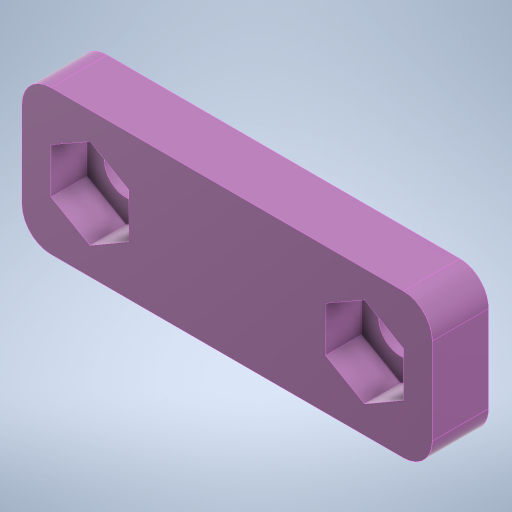
# Autodesk Inventor part: Крепежи динамиков
Saved by Autodesk Inventor 2024 (Build 280153020, 153B)
## iProperties
Created: 2023-06-10
Part Number: Крепежи динамиков
Material: Типовые
Document SubType Name: Modeling
Designer: Admin
Density: 1 g/cm^3
Appearance: По умолчанию
Author: Admin
Autodesk Inventor part; units mm, degrees
ref_plane "YZ Plane" through (0, 0, 0) normal (1, 0, 0) x (0, 1, 0)
ref_plane "XZ Plane" through (0, 0, 0) normal (0, 1, 0) x (-1, 0, 0)
ref_plane "XY Plane" through (0, 0, 0) normal (0, 0, 1) x (1, 0, 0)
sketch "Эскиз1" plane through (0, 0, 0) normal (0, 0, 1) x (1, 0, 0)
  line L0 (-6.8, -1.5588) -> (-9.5, -3.1177)
  line L1 (-9.5, -3.1177) -> (-12.2, -1.5588)
  circle A0 centre (-9.5, 0) radius 1.5
  line L2 (-6.8, 1.5588) -> (-6.8, -1.5588)
  line L3 (-12.2, -1.5588) -> (-12.2, 1.5588)
  line L4 (-9.5, 3.1177) -> (-6.8, 1.5588)
  line L5 (-12.2, 1.5588) -> (-9.5, 3.1177)
  line L6 (6.8, -1.5588) -> (6.8, 1.5588)
  line L7 (6.8, 1.5588) -> (9.5, 3.1177)
  line L8 (9.5, -3.1177) -> (6.8, -1.5588)
  circle A1 centre (9.5, 0) radius 1.5
  line L9 (9.5, 3.1177) -> (12.2, 1.5588)
  line L10 (12.2, 1.5588) -> (12.2, -1.5588)
  line L11 (12.2, -1.5588) -> (9.5, -3.1177)
  line L12 (-12.2, 5) -> (12.2, 5)
  line L13 (14.2, 3) -> (14.2, -3)
  line L14 (12.2, -5) -> (-12.2, -5)
  line L15 (-14.2, -3) -> (-14.2, 3)
  arc A2 (-12.2, 5) -> (-14.2, 3) centre (-12.2, 3) ccw
  arc A3 (-14.2, -3) -> (-12.2, -5) centre (-12.2, -3) ccw
  arc A4 (12.2, -5) -> (14.2, -3) centre (12.2, -3) ccw
  arc A5 (14.2, 3) -> (12.2, 5) centre (12.2, 3) ccw
  line L16 (0, 0) -> (0, 2.3671) construction
  point P0 (14.2, 0)
  point P1 (-14.2, 0)
  point P2 (0, 5)
  dimension "Width" = 10
  dimension "d6" = 2
  dimension "d12" = 13.6
  constraints: 34 end point, 8 point on circle, 8 tangent, 6 centre point, 5 parallel, 4 equal radius, 3 coincident, 3 horizontal alignment, 3 midpoint, 3 vertical, 1 horizontal, 1 perpendicular, 1 vertical alignment, 28 other
  measures "Width" distance between parallel lines of L14 L12
  measures "d6" radius of A2
  measures "d12" distance between parallel lines of L6 L2
extrude "Выдавливание1" add sketch "Эскиз1" against normal blind 1.5 contours L0 L1 L3 L5 L4 L2 | L6 L7 L9 L10 L11 L8 | L12 A5 L13 A4 L14 A3 L15 A2
extrude "Выдавливание2" add sketch "Эскиз1" along normal blind 2.5 contours L12 A5 L13 A4 L14 A3 L15 A2
chamfer "Фаска1" distance 0.3 distance2 0.1 8 edges at (0, 5, -1.5) (13.6142, 4.4142, -1.5) (14.2, 0, -1.5) (13.6142, -4.4142, -1.5) (0, -5, -1.5) (-13.6142, -4.4142, -1.5) (-14.2, 0, -1.5) (-13.6142, 4.4142, -1.5) measured on face at (2.8826, -3.7448, -1.5)
equation "\"d8\" = Thick - Nut_thick"
equation "\"Thick\" = 4"
equation "\"Nut_thick\" = 2.5"
